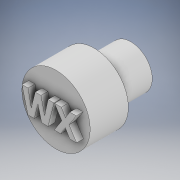
# Autodesk Inventor part: IPC WX key
Saved by Autodesk Inventor 2022 (Build 260153000, 153)
## iProperties
Created: 2022-01-01
Part Number: IPC WX key
Material: Generic
Document SubType Name: Modeling
Designer: solor
Density: 1 g/cm^3
Appearance: Default
Author: solor
Autodesk Inventor part; units mm, degrees
ref_plane "YZ Plane" through (0, 0, 0) normal (1, 0, 0) x (0, 1, 0)
ref_plane "XZ Plane" through (0, 0, 0) normal (0, 1, 0) x (-1, 0, 0)
ref_plane "XY Plane" through (0, 0, 0) normal (0, 0, 1) x (1, 0, 0)
sketch "Sketch1" plane through (0, 0, 0) normal (0, 0, 1) x (1, 0, 0)
  circle A0 centre (0, 0) radius 2.8
  line L0 (-0.675, 0.675) -> (-0.675, 2.025)
  line L1 (-0.675, 2.025) -> (0.675, 2.025)
  line L2 (0.675, 2.025) -> (0.675, 0.675)
  line L3 (0.675, 0.675) -> (2.025, 0.675)
  line L4 (2.025, 0.675) -> (2.025, -0.675)
  line L5 (2.025, -0.675) -> (0.675, -0.675)
  line L6 (0.675, -0.675) -> (0.675, -2.025)
  line L7 (0.675, -2.025) -> (-0.675, -2.025)
  line L8 (-0.675, -2.025) -> (-0.675, -0.675)
  line L9 (-0.675, -0.675) -> (-2.025, -0.675)
  line L10 (-2.025, -0.675) -> (-2.025, 0.675)
  line L11 (-2.025, 0.675) -> (-0.675, 0.675)
  circle A1 centre (0, 0) radius 4.94 construction
  circle A2 centre (0, 0) radius 4.47
  point P0 (-6.07, -6.1)
  dimension "d16" = 9.88
  dimension "d17" = 0.47
  constraints: 24 end point, 3 centre point, 1 coincident
  measures "d16" diameter of A1
  measures "d17" radial gap between concentric circles of A1 A2
extrude "Extrusion8" add sketch "Sketch1" along normal blind 5 contours A0 | L0 L1 L2 L3 L4 L5 L6 L7 L8 L9 L10 L11 | A2
extrude "Extrusion9" add sketch "Sketch1" against normal blind 4.8 contours A0
sketch "Sketch4" plane through (0, 0, 5) normal (0, 0, 1) x (1, 0, 0)
  line L0 (-3.616, 1.525) -> (3.616, 1.525) construction
  line L1 (3.616, 1.525) -> (3.616, -1.525) construction
  line L2 (3.616, -1.525) -> (-3.616, -1.525) construction
  line L3 (-3.616, -1.525) -> (-3.616, 1.525) construction
  line L4 (0.6327, 1.525) -> (-0.1384, -1.525)
  line L5 (-0.1384, -1.525) -> (-0.9788, -1.525)
  line L6 (-0.9788, -1.525) -> (-1.4682, 0.3609)
  line L7 (-1.4682, 0.3609) -> (-1.9402, -1.525)
  line L8 (-1.9402, -1.525) -> (-2.7831, -1.525)
  line L9 (-2.7831, -1.525) -> (-3.5542, 1.525)
  line L10 (-3.5542, 1.525) -> (-2.7583, 1.525)
  line L11 (-2.7583, 1.525) -> (-2.3382, -0.5166)
  line L12 (-2.3382, -0.5166) -> (-1.829, 1.525)
  line L13 (-1.829, 1.525) -> (-1.0677, 1.525)
  line L14 (-1.0677, 1.525) -> (-0.5833, -0.519)
  line L15 (-0.5833, -0.519) -> (-0.1434, 1.525)
  line L16 (-0.1434, 1.525) -> (0.6327, 1.525)
  line L17 (3.5913, -1.525) -> (2.7064, -1.525)
  line L18 (2.7064, -1.525) -> (2.1182, -0.5536)
  line L19 (2.1182, -0.5536) -> (1.5176, -1.525)
  line L20 (1.5176, -1.525) -> (0.6698, -1.525)
  line L21 (0.6698, -1.525) -> (1.6609, 0.0099)
  line L22 (1.6609, 0.0099) -> (0.7094, 1.525)
  line L23 (0.7094, 1.525) -> (1.5942, 1.525)
  line L24 (1.5942, 1.525) -> (2.1454, 0.6031)
  line L25 (2.1454, 0.6031) -> (2.7114, 1.525)
  line L26 (2.7114, 1.525) -> (3.5592, 1.525)
  line L27 (3.5592, 1.525) -> (2.6026, 0.042)
  line L28 (2.6026, 0.042) -> (3.5913, -1.525)
  point P0 (0, 0)
  point P1 (0, -1.525)
  point P2 (3.616, 0)
  point P3 (0, 0)
  point P4 (0, 0)
  constraints: 2 midpoint, 1 coincident, 2 other
extrude "Extrusion10" add sketch "Sketch4" along normal blind 0.9
body "Solid2"
